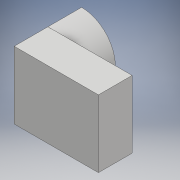
# Autodesk Inventor part: 39
Saved by Autodesk Inventor 2017 (Build 210142000, 142)
## iProperties
Part Number: 39
Material: 一般
Document SubType Name: Modeling
Designer: Brian
Density: 1 g/cm^3
Appearance: 預設
Mass: 60.2832 g
Surface Area: 101.494 cm^2
Volume: 60.2832 cm^3
Author: Brian
Autodesk Inventor part; units mm, degrees
ref_plane "YZ Plane" through (0, 0, 0) normal (1, 0, 0) x (0, 1, 0)
ref_plane "XZ Plane" through (0, 0, 0) normal (0, 1, 0) x (-1, 0, 0)
ref_plane "XY Plane" through (0, 0, 0) normal (0, 0, 1) x (1, 0, 0)
sketch "草圖1" plane through (0, 0, 0) normal (0, 1, 0) x (-1, 0, 0)
  line L0 (0, 0) -> (-50, 0)
  line L1 (-50, 0) -> (-50, -40)
  line L2 (-50, -40) -> (0, -40)
  line L3 (0, -40) -> (0, 0)
  dimension "d0" = 40
  dimension "d1" = 50
  constraints: 8 end point, 2 parallel, 1 horizontal, 1 perpendicular
  measures "d0" distance of L2.end L0.start
  measures "d1" distance of L1.end L2.end
extrude "擠出1" add sketch "草圖1" along normal blind 20
sketch "草圖2" plane through (0, 20, 0) normal (0, 1, 0) x (1, 0, 0)
  line L0 (0, 0) -> (20, 0)
  line L1 (20, 0) -> (20, 40)
  line L2 (20, 40) -> (0, 40)
  line L3 (0, 40) -> (0, 0)
  dimension "d4" = 40
  dimension "d5" = 20
  constraints: 8 end point, 2 parallel, 1 horizontal, 1 perpendicular
  measures "d4" distance of L0.end L1.end
  measures "d5" distance between parallel lines of L3 L1
extrude "擠出2" add sketch "草圖2" along normal blind 20
fillet "圓角1" radius 20 1 edges at (20, 30, 0)
sketch "草圖3" plane through (50, 0, -40) normal (0, 0, -1) x (-1, 0, 0)
  line L0 (30, 40) -> (50, 40) projected
  line L1 (0, 20) -> (30, 20) projected
  line L2 (30, 40) -> (0, 20)
  line L3 (0, 20) -> (30, 20)
  line L4 (30, 20) -> (30, 40)
  point P0 (50, 0)
  constraints: 6 end point, 1 collinear, 1 perpendicular
extrude "擠出3" add sketch "草圖3" against normal blind 20
